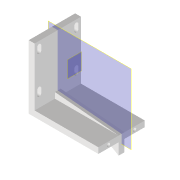
# Autodesk Inventor part: 40_XYZstage_micrometer_motorized_nema8_lightsheet_samplemount_ontop
Saved by Autodesk Inventor 2022 (Build 260153000, 153)
## iProperties
Created: 2023-07-30
Part Number: 40_XYZstage_micrometer_motorized_nema8_lightsheet_samplemount_ontop
Material: Generisch
Document SubType Name: Modeling
Designer: diederichbenedict
Density: 1 g/cm^3
Appearance: Vorgabe
Author: diederichbenedict
Autodesk Inventor part; units mm, degrees
ref_plane "YZ Plane" through (0, 0, 0) normal (1, 0, 0) x (0, 1, 0)
ref_plane "XZ Plane" through (0, 0, 0) normal (0, 1, 0) x (-1, 0, 0)
ref_plane "XY Plane" through (0, 0, 0) normal (0, 0, 1) x (1, 0, 0)
ref_plane "Arbeitsebene1" through (-0.5, 64.1414, -11) normal (-1, 0, 0) x (0, 0, 1)
sketch "Skizze1" plane through (-0.5, 64.1414, -11) normal (-1, 0, 0) x (0, 0, 1)
  line L0 (40, -27) -> (40, -40) projected
  line L1 (40, -27) -> (29, -27) projected
  line L2 (29, -40) -> (29, -27) projected
  line L3 (29, -40) -> (40, -40) projected
  circle A0 centre (32, -32) radius 1.5 projected
  circle A1 centre (36, -36) radius 1.75 projected
  line L4 (0, -40) -> (11, -40) projected
  line L5 (11, -40) -> (11, -27) projected
  line L6 (0, -27) -> (11, -27) projected
  line L7 (0, -27) -> (0, -40) projected
  circle A2 centre (8, -32) radius 1.5 projected
  circle A3 centre (4, -36) radius 1.75 projected
  line L8 (0, 0) -> (0, -13) projected
  line L9 (0, -13) -> (11, -13) projected
  line L10 (11, 0) -> (11, -13) projected
  line L11 (0, 0) -> (11, 0) projected
  circle A4 centre (8, -8) radius 1.5 projected
  circle A5 centre (4, -4) radius 1.75 projected
  line L12 (29, 0) -> (40, 0) projected
  line L13 (29, 0) -> (29, -13) projected
  line L14 (40, -13) -> (29, -13) projected
  line L15 (40, 0) -> (40, -13) projected
  circle A6 centre (32, -8) radius 1.5 projected
  circle A7 centre (36, -4) radius 1.75 projected
  line L16 (40, -40) -> (0, -40)
  line L17 (0, -40) -> (0, 0)
  line L18 (0, 0) -> (40, 0)
  line L19 (40, 0) -> (40, -40)
  line L20 (40, -40) -> (0, -40)
  line L21 (0, -40) -> (0, -55)
  line L22 (0, -55) -> (40, -55)
  line L23 (40, -55) -> (40, -40)
  line L24 (36, -36) -> (36, -40) construction
  line L25 (37.75, -36) -> (37.75, -40)
  line L26 (34.25, -40) -> (34.25, -36)
  arc A8 (37.75, -36) -> (34.25, -36) centre (36, -36) ccw
  arc A9 (34.25, -40) -> (37.75, -40) centre (36, -40) ccw
  line L27 (4, -36) -> (4, -40) construction
  line L28 (5.75, -36) -> (5.75, -40)
  line L29 (2.25, -40) -> (2.25, -36)
  arc A10 (5.75, -36) -> (2.25, -36) centre (4, -36) ccw
  arc A11 (2.25, -40) -> (5.75, -40) centre (4, -40) ccw
  line L30 (4, -4) -> (4, -8) construction
  line L31 (5.75, -4) -> (5.75, -8)
  line L32 (2.25, -8) -> (2.25, -4)
  arc A12 (5.75, -4) -> (2.25, -4) centre (4, -4) ccw
  arc A13 (2.25, -8) -> (5.75, -8) centre (4, -8) ccw
  line L33 (36, -4) -> (36, -8) construction
  line L34 (37.75, -4) -> (37.75, -8)
  line L35 (34.25, -8) -> (34.25, -4)
  arc A14 (37.75, -4) -> (34.25, -4) centre (36, -4) ccw
  arc A15 (34.25, -8) -> (37.75, -8) centre (36, -8) ccw
  point P0 (11, -64.1414)
  point P1 (40, -13)
  point P2 (0, -13)
  point P3 (0, -27)
  point P4 (0, -40)
  point P5 (36, -38)
  point P6 (4, -38)
  point P7 (4, -6)
  point P8 (36, -6)
  point P9 (37.75, -4)
  point P10 (34.25, -4)
  point P11 (5.75, -4)
  point P12 (2.25, -4)
  dimension "d0" = 15
  constraints: 48 end point, 16 point on circle, 16 tangent, 8 centre point, 8 parallel, 4 midpoint, 4 point on line, 3 perpendicular, 2 concentric, 2 horizontal, 1 vertical
  measures "d0" distance of L21.end L20.end
extrude "Extrusion1" add sketch "Skizze1" along normal blind 5 contours L0 L3 L25 A1 L26 L2 L1 | L1 L2 L16 L5 L6 L17 L9 L10 L18 L13 L14 L19 | L23 L22 L21 L4 A11 L16 L3 A9 | L14 L13 L12 L15 | L4 L28 A3 L29 L7 L6 L5 | L10 L9 L8 L11 | A0 | A2 | A4 | A6
sketch "Skizze2" plane through (-0.5, 64.1414, -11) normal (1, 0, 0) x (0, 0, -1)
  line L0 (-40, -55) -> (-40, 0) projected
  line L1 (0, -55) -> (-40, -55) projected
  line L2 (0, 0) -> (0, -55) projected
  line L3 (-40, 0) -> (0, 0) projected
  arc A0 (-2.25, -36) -> (-5.75, -36) centre (-4, -36) ccw projected
  arc A1 (-2.25, -4) -> (-5.75, -4) centre (-4, -4) ccw projected
  arc A2 (-34.25, -4) -> (-37.75, -4) centre (-36, -4) ccw projected
  arc A3 (-34.25, -36) -> (-37.75, -36) centre (-36, -36) ccw projected
  line L4 (0, -55) -> (-40, -55)
  line L5 (-40, -55) -> (-40, -50)
  line L6 (-40, -50) -> (0, -50)
  line L7 (0, -50) -> (0, -55)
  line L8 (-2.25, -40) -> (-2.25, -36) projected
  arc A4 (-5.75, -40) -> (-2.25, -40) centre (-4, -40) ccw projected
  line L9 (-5.75, -36) -> (-5.75, -40) projected
  line L10 (-37.75, -4) -> (-37.75, -8) projected
  line L11 (-34.25, -8) -> (-34.25, -4) projected
  arc A5 (-37.75, -8) -> (-34.25, -8) centre (-36, -8) ccw projected
  line L12 (-34.25, -40) -> (-34.25, -36) projected
  arc A6 (-37.75, -40) -> (-34.25, -40) centre (-36, -40) ccw projected
  line L13 (-37.75, -36) -> (-37.75, -40) projected
  line L14 (-5.75, -4) -> (-5.75, -8) projected
  line L15 (-2.25, -8) -> (-2.25, -4) projected
  arc A7 (-5.75, -8) -> (-2.25, -8) centre (-4, -8) ccw projected
  point P0 (-11, -64.1414)
  dimension "d3" = 5
  constraints: 8 end point, 2 parallel, 1 horizontal, 1 perpendicular, 1 point on line
  measures "d3" distance of L4.end L5.end
extrude "Extrusion2" add sketch "Skizze2" along normal blind 55 contours L0 L6 L2 L1
ref_plane "Arbeitsebene2" through (-0.5, 64.1414, 9) normal (0, 0, -1) x (-1, 0, 0)
sketch "Skizze3" plane through (-0.5, 64.1414, 9) normal (0, 0, -1) x (-1, 0, 0)
  line L0 (0, 0) -> (0, -50) projected
  line L1 (0, -50) -> (-55, -50) projected
  line L2 (-55, -55) -> (-55, -50) projected
  line L3 (5, -55) -> (-55, -55) projected
  line L4 (5, 0) -> (5, -55) projected
  line L5 (0, 0) -> (5, 0) projected
  line L6 (0, -50) -> (-55, -50) projected
  line L7 (-55, -50) -> (0, -45)
  line L8 (-55, -55) -> (-55, -50) projected
  line L9 (-55, -55) -> (-55, -63)
  line L10 (-55, -63) -> (-41.1436, -55)
  line L11 (-55, -55) -> (5, -55) projected
  line L12 (-41.1436, -55) -> (-55, -55)
  line L13 (-55, -50) -> (-55, -47.5)
  line L14 (-55, -47.5) -> (-37.6795, -48.4254)
  point P0 (-0.5, -64.1414)
  point P1 (-41.1436, -55)
  dimension "d7" = 5
  dimension "d14" = 8
  dimension "d15" = 60
  constraints: 12 end point, 2 point on line, 2 vertical, 1 collinear
  measures "d7" distance from line of L1 L7.end
  measures "d14" distance of L2.start L9.end
  measures "d15" angle of L10 L9
extrude "Extrusion3" add sketch "Skizze3" along normal mid plane 5 contours L0 L1 L7 | L7 L13 L14 | L10 L9 L3
sketch "Skizze4" plane through (54.5, 64.1414, -11) normal (1, 0, 0) x (0, 0, -1)
  line L0 (-40, -50) -> (-40, -55) projected
  line L1 (-40, -55) -> (-22.5, -55) projected
  line L2 (0, -55) -> (0, -50) projected
  line L3 (-22.5, -50) -> (-40, -50) projected
  line L4 (0, -50) -> (-17.5, -50) projected
  circle A0 centre (-8.75, -52.5) radius 1.4
  circle A1 centre (-31.25, -52.5) radius 1.4
  line L5 (-22.5, -63) -> (-22.5, -55) projected
  line L6 (-17.5, -63) -> (-22.5, -63) projected
  line L7 (-17.5, -55) -> (-17.5, -63) projected
  line L8 (-17.5, -55) -> (0, -55) projected
  line L9 (-17.5, -47.5) -> (-17.5, -50) projected
  line L10 (-22.5, -47.5) -> (-17.5, -47.5) projected
  line L11 (-22.5, -50) -> (-22.5, -47.5) projected
  point P0 (-11, -64.1414)
  dimension "d10" = 2.8
  dimension "d11" = 2.8
  constraints: 2 centre point
  measures "d10" diameter of A0
  measures "d11" diameter of A1
extrude "Extrusion4" cut sketch "Skizze4" against normal through all contours A0 | A1
